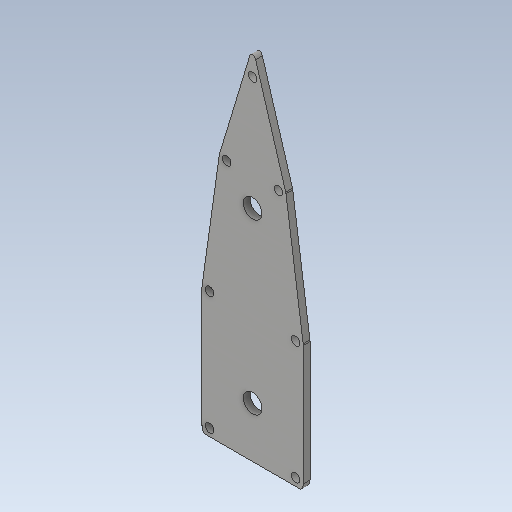
# Autodesk Inventor part: bund vange-endeplade
Saved by Autodesk Inventor 2020.1 (Build 241239000, 239)
## iProperties
Created: 2019-09-26
Part Number: bund vange-endeplade
Material: S235JR
Document SubType Name: Sheet Metal
Designer: loppen
Density: 7.85 g/cm^3
Sheet Metal Rule: Default_mm
Appearance: Light Gray
Mass: 2276.68 g
Surface Area: 831.189 cm^2
Volume: 290.024 cm^3
Flat Pattern Width: 13.8954 cm
Flat Pattern Length: 42.1731 cm
Flat Pattern Area: 586.012 cm^2
Sheet Metal Width: 138,954 mm
Sheet Metal Length: 421,731 mm
Sheet Metal Area: 58601,168 mm^2
Author: loppen
Autodesk Inventor part; units mm, degrees
ref_plane "YZ Plane" through (0, 0, 0) normal (1, 0, 0) x (0, 1, 0)
ref_plane "XZ Plane" through (0, 0, 0) normal (0, 1, 0) x (-1, 0, 0)
ref_plane "Work Plane1" through (0, 0, 0) normal (0, 0, 1) x (1, 0, 0)
sketch "Sketch1" plane through (0, 0, 0) normal (0, 0, 1) x (1, 0, 0)
  line L0 (-65.5, -425.0611) -> (-65.5, -432.1593)
  line L1 (-120, -425.0611) -> (-65.5, -425.0611)
  ellipse E0 centre (-120, -417.963) end of major axis (-120, -425.0611) minor radius 4 (-124, -417.963) -> (-120, -425.0611) ccw
  line L2 (-124, -275.99) -> (-124, -417.963)
  ellipse E1 centre (-120, -275.99) end of major axis (-120, -268.8918) minor radius 4 (-123.8796, -274.2613) -> (-124, -275.99) ccw
  line L3 (-103.5409, -130.5299) -> (-123.8796, -274.2613)
  ellipse E2 centre (-99.6613, -132.2586) end of major axis (-99.6613, -125.1604) minor radius 4 (-103.1868, -128.9053) -> (-103.5409, -130.5299) ccw
  line L4 (-67.5255, -10.843) -> (-103.1868, -128.9053)
  ellipse E3 centre (-64, -14.1963) end of major axis (-64, -7.0982) minor radius 4 (-60.4745, -10.843) -> (-67.5255, -10.843) ccw
  line L5 (-24.8132, -128.9053) -> (-60.4745, -10.843)
  ellipse E4 centre (-28.3387, -132.2586) end of major axis (-28.3387, -125.1604) minor radius 4 (-24.4591, -130.5299) -> (-24.8132, -128.9053) ccw
  line L6 (-4.1204, -274.2613) -> (-24.4591, -130.5299)
  ellipse E5 centre (-8, -275.99) end of major axis (-8, -268.8918) minor radius 4 (-4, -275.99) -> (-4.1204, -274.2613) ccw
  line L7 (-4, -417.963) -> (-4, -275.99)
  ellipse E6 centre (-8, -417.963) end of major axis (-8, -425.0611) minor radius 4 (-8, -425.0611) -> (-4, -417.963) ccw
  line L8 (-62.5, -425.0611) -> (-8, -425.0611)
  line L9 (-62.5, -432.1593) -> (-62.5, -425.0611)
  line L10 (-8, -432.1593) -> (-62.5, -432.1593)
  ellipse E7 centre (-8, -417.963) end of major axis (-8, -432.1593) minor radius 8 (-8, -432.1593) -> (0, -417.963) ccw
  line L11 (0, -275.99) -> (0, -417.963)
  ellipse E8 centre (-8, -275.99) end of major axis (-8, -261.7937) minor radius 8 (0, -275.99) -> (-0.2409, -272.5326) ccw
  line L12 (-20.5796, -128.8012) -> (-0.2409, -272.5326)
  ellipse E9 centre (-28.3387, -132.2586) end of major axis (-28.3387, -118.0623) minor radius 8 (-20.5796, -128.8012) -> (-21.2877, -125.5519) ccw
  line L13 (-56.949, -7.4896) -> (-21.2877, -125.5519)
  ellipse E10 centre (-64, -14.1963) end of major axis (-64, 0) minor radius 8 (-56.949, -7.4896) -> (-71.051, -7.4896) ccw
  line L14 (-106.7123, -125.5519) -> (-71.051, -7.4896)
  ellipse E11 centre (-99.6613, -132.2586) end of major axis (-99.6613, -118.0623) minor radius 8 (-106.7123, -125.5519) -> (-107.4204, -128.8012) ccw
  line L15 (-127.7591, -272.5326) -> (-107.4204, -128.8012)
  ellipse E12 centre (-120, -275.99) end of major axis (-120, -261.7937) minor radius 8 (-127.7591, -272.5326) -> (-128, -275.99) ccw
  line L16 (-128, -417.963) -> (-128, -275.99)
  ellipse E13 centre (-120, -417.963) end of major axis (-120, -432.1593) minor radius 8 (-128, -417.963) -> (-120, -432.1593) ccw
  line L17 (-65.5, -432.1593) -> (-120, -432.1593)
  line L18 (-62.5, -425.0611) -> (-65.5, -425.0611)
  point P0 (0, 0)
extrude "Plate1" add sketch "Sketch1" along normal blind 8 contours L1 E0 L2 E1 L3 E2 L4 E3 L5 E4 L6 E5 L7 E6 L8 L18
sketch "Sketch2" plane through (0, 0, 8) normal (0, 0, 1) x (1, 0, 0)
  line L0 (-8, -425.0611) -> (-120, -425.0611) projected
  ellipse E0 centre (-8, -417.963) end of major axis (-8, -425.0611) minor radius 4 (-8, -425.0611) -> (-4, -417.963) ccw projected
  line L1 (-4, -275.99) -> (-4, -417.963) projected
  ellipse E1 centre (-8, -275.99) end of major axis (-8, -268.8918) minor radius 4 (-4, -275.99) -> (-4.1204, -274.2613) ccw projected
  line L2 (-24.4591, -130.5299) -> (-4.1204, -274.2613) projected
  ellipse E2 centre (-28.3387, -132.2586) end of major axis (-28.3387, -125.1604) minor radius 4 (-24.4591, -130.5299) -> (-24.8132, -128.9053) ccw projected
  line L3 (-60.4745, -10.843) -> (-24.8132, -128.9053) projected
  ellipse E3 centre (-64, -14.1963) end of major axis (-64, -7.0982) minor radius 4 (-60.4745, -10.843) -> (-67.5255, -10.843) ccw projected
  line L4 (-103.1868, -128.9053) -> (-67.5255, -10.843) projected
  ellipse E4 centre (-99.6613, -132.2586) end of major axis (-99.6613, -125.1604) minor radius 4 (-103.1868, -128.9053) -> (-103.5409, -130.5299) ccw projected
  line L5 (-123.8796, -274.2613) -> (-103.5409, -130.5299) projected
  ellipse E5 centre (-120, -275.99) end of major axis (-120, -268.8918) minor radius 4 (-123.8796, -274.2613) -> (-124, -275.99) ccw projected
  line L6 (-124, -417.963) -> (-124, -275.99) projected
  ellipse E6 centre (-120, -417.963) end of major axis (-120, -425.0611) minor radius 4 (-124, -417.963) -> (-120, -425.0611) ccw projected
  line L7 (-64, -470.7435) -> (-64, 33.682) construction
  line L8 (-8, -425.0611) -> (-120, -425.0611) construction
  circle A0 centre (-64, -365.0611) radius 11
  circle A1 centre (-64, -165.0611) radius 11
  circle A2 centre (-115, -416.0611) radius 5
  circle A3 centre (-115, -275.746) radius 5
  circle A4 centre (-94.6057, -131.6217) radius 5
  circle A5 centre (-64, -30.2968) radius 5
  circle A6 centre (-33.3943, -131.6217) radius 5
  circle A7 centre (-13, -275.746) radius 5
  circle A8 centre (-13, -416.0611) radius 5
  point P0 (0, 0)
  dimension "d1" = 22
  dimension "d2" = 22
  dimension "d3" = 10
  dimension "d4" = 10
  dimension "d5" = 10
  dimension "d7" = 10
  dimension "d9" = 10
  dimension "d11" = 10
  dimension "d13" = 10
  dimension "d15" = 9
  dimension "d16" = 9
  dimension "d17" = 4
  dimension "d18" = 9
  dimension "d19" = 9
  dimension "d20" = 9
  dimension "d21" = 9
  dimension "d22" = 9
  dimension "d23" = 9
  dimension "d24" = 9
  dimension "d25" = 9
  dimension "d26" = 9
  dimension "d27" = 9
  dimension "d28" = 9
  dimension "d29" = 9
  dimension "d30" = 60
  dimension "d31" = 60
  dimension "d33" = 200
  constraints: 9 centre point, 3 point on line, 2 end point, 1 perpendicular, 7 other
  measures "d1" diameter of A0
  measures "d2" diameter of A1
  measures "d3" diameter of A2
  measures "d4" diameter of A3
  measures "d5" diameter of A4
  measures "d7" diameter of A5
  measures "d9" diameter of A6
  measures "d11" diameter of A7
  measures "d13" diameter of A8
  measures "d15" distance from line of A2.centre L6
  measures "d16" distance from line of A2.centre L0
  measures "d17" distance edge to line of A2 L6
  measures "d18" distance from line of A3.centre L6
  measures "d19" distance from line of A3.centre L5
  measures "d20" distance from line of A4.centre L5
  measures "d21" distance from line of A4.centre L4
  measures "d22" distance from line of A5.centre L4
  measures "d23" distance from line of A5.centre L3
  measures "d24" distance from line of A6.centre L3
  measures "d25" distance from line of A6.centre L2
  measures "d26" distance from line of A7.centre L2
  measures "d27" distance from line of A7.centre L1
  measures "d28" distance from line of A8.centre L1
  measures "d29" distance from line of A8.centre L0
  measures "d30" distance between parallel lines of L1 L7
  measures "d31" distance from line of L0 A0.centre
  measures "d33" distance of A0.centre A1.centre
extrude "zinkdrænshuller" cut sketch "Sketch2" against normal blind 8 contours A0 | A1 | A2 | A3 | A4 | A5 | A6 | A7 | A8
equation "\"d2\" = d1"
equation "\"d4\" = d3"
equation "\"d5\" = d6"
equation "\"d7\" = d8"
equation "\"d9\" = d10"
equation "\"d11\" = d12"
equation "\"d13\" = d14"
equation "\"d16\" = d15"
equation "\"d18\" = d16"
equation "\"d19\" = d16"
equation "\"d20\" = d16"
equation "\"d21\" = d16"
equation "\"d22\" = d16"
equation "\"d23\" = d16"
equation "\"d24\" = d16"
equation "\"d25\" = d16"
equation "\"d26\" = d16"
equation "\"d27\" = d16"
equation "\"d28\" = d16"
equation "\"d29\" = d16"
equation "\"d31\" = d30"
equation "\"d34\" = Thickness"
equation "\"d0\" = Thickness"
equation "\"BendRadius\" = Thickness"
equation "\"BendReliefWidth\" = Thickness"
equation "\"BendReliefDepth\" = 0.5 * Thickness"
equation "\"CornerReliefSize\" = 4 * Thickness"
equation "\"MinimumRemnant\" = 2 * Thickness"
equation "\"TransitionRadius\" = BendRadius"
equation "\"JacobiRadiusSize\" = BendRadius"
equation "\"GapSize\" = Thickness"
equation "\"d6\" = 10"
equation "\"d8\" = 10"
equation "\"d10\" = 10"
equation "\"d12\" = 10"
equation "\"d14\" = 10"
equation "\"Thickness\" = 8"
body "Solid1"
